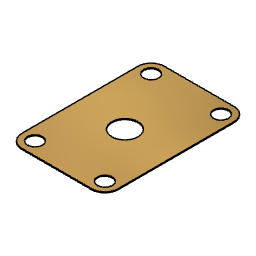
front cover v4 (Autodesk Fusion 360 design; units mm, degrees)
Autodesk Fusion 360 part; units mm, degrees
note: some values were not read from the file. Set by a fixed rule: the direction of a hole.
sketch "Sketch1" plane through (0, 0, 0) normal (0, 1, 0) x (1, 0, 0)
  line L0 (0, 0) -> (11, 0)
  line L1 (11, 0) -> (11, -16.3)
  line L2 (11, -16.3) -> (0, -16.3)
  line L3 (0, -16.3) -> (0, 0)
  line L4 (1.5, -14.8) -> (1.5, -1.5) construction
  line L5 (1.5, -1.5) -> (9.5, -1.5) construction
  line L6 (9.5, -1.5) -> (9.5, -14.8) construction
  line L7 (9.5, -14.8) -> (1.5, -14.8) construction
  circle A0 centre (5.5, -8.5) radius 1.5
  line L8 (5.5, -14.8) -> (5.5, -8.5) construction
  point P0 (1.5, -1.5)
  point P1 (9.5, -1.5)
  point P2 (9.5, -14.8)
  point P3 (1.5, -14.8)
  dimension "d1" = 16.3
  dimension "d2" = 11
  dimension "d3" = 1.5
  dimension "d4" = 6.3
  dimension "d5" = 3
  constraint horizontal L0
  constraint vertical L1
  constraint horizontal L2
  constraint vertical L3
  constraint coincident L0.start L3.end
  constraint coincident P0 L4.end
  constraint coincident P1 L5.end
  constraint coincident P2 L6.end
  constraint coincident P3 L4.start
  constraint midpoint L7 L8.start
  constraint coincident A0.centre L8.end
  constraint vertical L8
  measures "d1" distance of L0.start L2.end
  measures "d2" distance of L0.start L0.end
  measures "d4" distance of L7 A0.centre
  measures "d5" diameter of A0
extrude "Extrude1" add sketch "Sketch1" along normal blind 0.1
hole "Hole1" at (1.5, 0, 14.8) at (1.5, 0, 1.5) at (9.5, 0, 1.5) at (9.5, 0, 14.8) direction (0, 1, 0) diameter 1.7 depth 12 tip angle 118
fillet "Fillet1" radius 1.5 4 edges at (11, 0.05, 16.3) (0, 0.05, 16.3) (0, 0.05, 0) (11, 0.05, 0)
equation "d1 = 11.3 mm + 5 mm"
equation "d2 = 8 mm + 3 mm"
